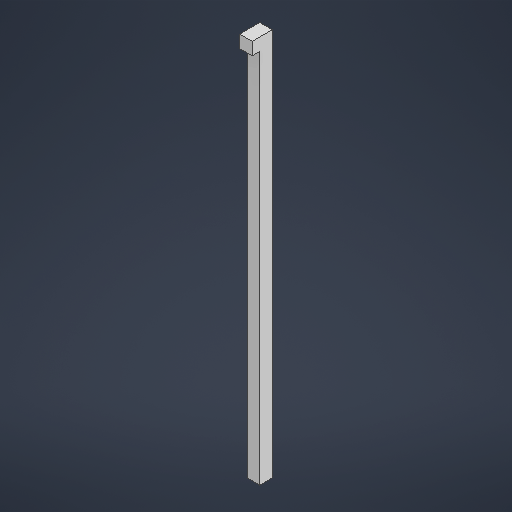
# Autodesk Inventor part: jst-ph-5p_wire
Saved by Autodesk Inventor 2025.2 (Build 292293000, 293)
## iProperties
Created: 2025-12-13
Part Number: jst-ph-5p_wire
Material: Generic
Document SubType Name: Modeling
Designer: sam
Density: 1 g/cm^3
Appearance: Default
Author: sam
Autodesk Inventor part; units mm, degrees
ref_plane "YZ Plane" through (0, 0, 0) normal (1, 0, 0) x (0, 1, 0)
ref_plane "XZ Plane" through (0, 0, 0) normal (0, 1, 0) x (-1, 0, 0)
ref_plane "XY Plane" through (0, 0, 0) normal (0, 0, 1) x (1, 0, 0)
sketch "Sketch1" plane through (0, 0, 0) normal (0, 1, 0) x (-1, 0, 0)
  line L0 (0.25, 0.25) -> (-0.25, 0.25)
  line L1 (-0.25, 0.25) -> (-0.25, -0.25)
  line L2 (-0.25, -0.25) -> (0.25, -0.25)
  line L3 (0.25, -0.25) -> (0.25, 0.25)
  line L4 (0.25, 0.25) -> (-0.25, -0.25) construction
  line L5 (-0.25, 0.25) -> (0.25, -0.25) construction
  point P0 (0, 0)
  dimension "d0" = 0.5
  dimension "d1" = 0.5
  constraints: 12 end point, 2 midpoint, 2 parallel, 1 horizontal, 1 perpendicular
  measures "d0" distance of L2.end L1.end
  measures "d1" distance of L1.end L0.end
extrude "Extrusion1" add sketch "Sketch1" along normal blind 15.45
sketch "Sketch2" plane through (-0.25, 0, 0.25) normal (0, 0, 1) x (1, 0, 0)
  line L0 (0, 0) -> (0, 15.45) projected
  line L1 (0.5, 0) -> (0.5, 15.45) projected
  line L2 (0, 15.45) -> (0.5, 15.45)
  line L3 (0.5, 15.45) -> (0.5, 14.95)
  line L4 (0.5, 14.95) -> (0, 14.95)
  line L5 (0, 14.95) -> (0, 15.45)
  point P0 (0.25, 0)
  point P1 (0, 14.95)
  dimension "d4" = 0.5
  constraints: 8 end point, 2 parallel, 1 horizontal, 1 perpendicular, 1 point on line
  measures "d4" distance of L2.end L3.end
extrude "Extrusion2" add sketch "Sketch2" along normal blind 0.3
body "Solid1"
